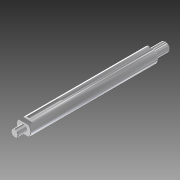
# Autodesk Inventor part: BB2-OutputShaft
Saved by Autodesk Inventor 2012 (Build 160160000, 160)
## iProperties
Company: FirstCadLibrary
Shininess: 64.0
Length Units: 11269
Angle Units: 11279
Time Units: 11290
Mass Units: 11283
Length Display Precision: 3
Angle Display Precision: 2
Compacted: True
Part Number: BB2-OutputShaft
Document SubType Name: Modeling
Created: 2007-01-08
Material: Steel, Mild
Designer: Ed Sparks
Catalog Web Link: www.banebots.com
Vendor: BaneBots
Mass: 123.935 g
Surface Area: 57.146 cm^2
Volume: 15.7678 cm^3
Density: 7.86 g/cm^3
Density: 0.0
Volumn: 0.0
Area: 0.0
PropertySet Name: Model Information
Control State: 0
Master: False
Checked Out: False
Author: Ed Sparks
Autodesk Inventor part; units mm, degrees
ref_plane "YZ Plane" through (0, 0, 0) normal (1, 0, 0) x (0, 1, 0)
ref_plane "XZ Plane" through (0, 0, 0) normal (0, 1, 0) x (-1, 0, 0)
sketch "Sketch1" plane through (0, 0, 0) normal (0, 0, 1) x (1, 0, 0)
  circle A0 centre (0, 0) radius 6.35
  dimension "d0" = 12.7
  constraints: 1 centre point, 1 coincident, 1 other
  measures "d0" diameter of A0
extrude "Extrusion1" add sketch "Sketch1" along normal mid plane 127
sketch "Sketch2" plane through (0, 0, 63.5) normal (0, 0, 1) x (1, 0, 0)
  circle A0 centre (0, 0) radius 6.35 projected
  line L0 (-4.5, 4.4802) -> (-4.5, -4.4802)
  line L1 (4.5, 4.4802) -> (4.5, -4.4802)
  line L2 (0, 0) -> (0, 6.1782) construction
  dimension "d3" = 9
  constraints: 6 end point, 4 point on circle, 2 vertical, 1 parallel, 1 other
  measures "d3" distance between parallel lines of L1 L0
extrude "Extrusion2" cut sketch "Sketch2" against normal blind 4 contours A0 L1 | L0 A0
sketch "Sketch3" plane through (0, 0, 63.5) normal (0, 0, 1) x (1, 0, 0)
  arc A0 (4.5, 4.4802) -> (-4.5, 4.4802) centre (0, 0) ccw projected
  circle A1 centre (0, 0) radius 3
  dimension "d6" = 6
  constraints: 1 centre point, 1 coincident, 1 concentric
  measures "d6" diameter of A1
extrude "Extrusion3" add sketch "Sketch3" along normal blind 8.2
chamfer "Chamfer1" distance 0.25 angle 45 4 edges at (-3, 0, 71.7) (0, -6.35, 63.5) (0, 6.35, 63.5) (-6.35, 0, -63.5)
ref_plane "Work Plane1" through (6.35, 0, 0) normal (1, 0, 0) x (0, 1, 0)
sketch "Sketch4" plane through (6.35, 0, 0) normal (1, 0, 0) x (0, 1, 0)
  line L0 (6.1, -63.5) -> (-6.1, -63.5) projected
  line L1 (0, -63.5) -> (0, -7.8695) construction
  line L2 (-1.5875, -63.5) -> (-1.5875, 30.1625)
  line L3 (0, 31.75) -> (0, 31.75)
  line L4 (1.5875, 30.1625) -> (1.5875, -63.5)
  arc A0 (0, 31.75) -> (-1.5875, 30.1625) centre (0, 30.1625) ccw
  arc A1 (1.5875, 30.1625) -> (0, 31.75) centre (0, 30.1625) ccw
  point P0 (1.5875, 31.75)
  dimension "d12" = 95.25
  dimension "d13" = 3.175
  dimension "d14" = 1.5875
  constraints: 8 end point, 4 point on circle, 4 point on line, 4 tangent, 3 perpendicular, 2 centre point, 1 concentric, 1 midpoint, 1 parallel, 1 other
  measures "d12" distance of point (1.587, 31.75) L4.end
  measures "d13" distance between parallel lines of L4 L2
  measures "d14" radius of A0
extrude "Extrusion4" cut sketch "Sketch4" against normal blind 1.5875
sketch "Sketch5" plane through (0, 0, -63.5) normal (0, 0, -1) x (-1, 0, 0)
  arc A0 (-5.8898, -1.5875) -> (-5.8898, 1.5875) centre (0, 0) ccw projected
  circle A1 centre (0, 0) radius 4
  circle A2 centre (0, 0) radius 6.35
  dimension "d18" = 8
  dimension "d19" = 12.7
  constraints: 2 centre point, 2 coincident
  measures "d18" diameter of A1
  measures "d19" diameter of A2
extrude "Extrusion5" cut sketch "Sketch5" against normal blind 12.7
chamfer "Chamfer2" distance 0.25 angle 45 3 edges at (4, 0, -63.5) (4, 0, -50.8) (-6.35, 0, -50.8)
body "Solid1"
